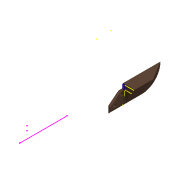
# Autodesk Inventor part: encoder guard mirror
Saved by Autodesk Inventor 2020 (Build 240168000, 168)
## iProperties
Created: 2020-01-15
Part Number: encoder guard mirror
Material: Bronze, Cast
Document SubType Name: Modeling
Designer: ball
Density: 8.87 g/cm^3
Appearance: Bronze - Satin
Mass: 40.1382 g
Surface Area: 24.9444 cm^2
Volume: 4.52517 cm^3
Author: ball
Autodesk Inventor part; units mm, degrees
ref_plane "YZ Plane" through (0, 0, 0) normal (1, 0, 0) x (0, 1, 0)
ref_plane "XZ Plane" through (0, 0, 0) normal (0, 1, 0) x (-1, 0, 0)
ref_plane "XY Plane" through (0, 0, 0) normal (0, 0, 1) x (1, 0, 0)
ref_plane "Work Plane6" through (0, 0, 0) normal (0, 0, 1) x (1, 0, 0)
sketch "Sketch1" plane through (0, 0, 0) normal (0, 0, 1) x (1, 0, 0)
  line L0 (25.4, -44.45) -> (0, -44.45) construction
  line L1 (25.4, -44.45) -> (12.7, -44.45)
  line L2 (12.7, -65.151) -> (25.4, -44.45)
  line L3 (12.7, -44.45) -> (12.7, -65.151)
  point P0 (0, 0)
  dimension "d0" = 20.701
  dimension "d1" = 12.7
  constraints: 6 end point, 1 midpoint, 1 perpendicular, 1 point on line
  measures "d0" distance from line of L0 L2.start
  measures "d1" distance from line of L1.start L3
revolve "Revolution1" add sketch "Sketch1" angle 180 mid plane about axis through (25.4, -44.45, 0) along (-1, 0, 0)
ref_plane "Work Plane10" through (12.7, -44.45, -31.115) normal (0, -1, 0) x (0, 0, -1)
sketch "Sketch2" plane through (12.7, -44.45, -31.115) normal (0, -1, 0) x (0, 0, -1)
  line L0 (0.635, -12.7) -> (0.635, 12.7) construction
  line L1 (9.525, 12.7) -> (-9.525, 12.7) construction
  line L2 (0.635, 0) -> (-31.115, 0)
  line L3 (-31.115, 0) -> (-31.115, 12.7)
  line L4 (-31.115, 12.7) -> (0.635, 12.7)
  line L5 (0.635, 12.7) -> (0.635, 0)
  point P0 (-31.115, -12.7)
  constraints: 8 end point, 2 parallel, 1 horizontal, 1 midpoint, 1 perpendicular
extrude "Extrusion1" add sketch "Sketch2" along normal blind 5.08
sketch "Sketch3" plane through (12.7, -49.53, -31.115) normal (0, -1, 0) x (1, 0, 0)
  point P0 (-12.7, 31.115)
ref_plane "Work Plane9" through (25.4, -44.45, -31.75) normal (0, 0, -1) x (-1, 0, 0)
sketch "Sketch4" plane through (25.4, -44.45, -31.75) normal (0, 0, -1) x (-1, 0, 0)
  line L0 (12.7, -5.08) -> (3.1166, -5.08)
  line L1 (0, 0) -> (12.7, -20.701) projected
  line L2 (12.7, -20.701) -> (12.7, 0) projected
  line L3 (12.7, -5.08) -> (12.7, -20.701)
  line L4 (12.7, -20.701) -> (3.1166, -5.08)
  point P0 (25.4, 44.45)
  constraints: 6 end point, 1 collinear, 1 horizontal, 1 point on line
extrude "Extrusion2" add sketch "Sketch4" against normal through all
ref_plane "Work Plane8" through (25.4, -47.625, 0) normal (0, 0, 1) x (1, 0, 0)
sketch "Sketch5" plane through (25.4, -47.625, 0) normal (0, 0, 1) x (1, 0, 0)
  line L0 (-12.7, 3.175) -> (0, 3.175) projected
  line L1 (-3.6741, -2.8138) -> (0, 3.175) projected
  line L2 (0, 3.175) -> (-3.6741, -2.8138)
  line L3 (-3.6741, -2.8138) -> (0, -4.7625)
  line L4 (0, -4.7625) -> (4.0347, 1.814)
  line L5 (4.0347, 1.814) -> (0, 3.175)
  point P0 (-25.4, 47.625)
  constraints: 8 end point, 1 collinear, 1 parallel
extrude "Extrusion3" cut sketch "Sketch5" against normal through all
sketch "Sketch6" plane through (12.7, -44.45, 20.701) normal (0, 1, 0) x (1, 0, 0)
  line L0 (0, 0) -> (0, 52.451) projected
  point P0 (-12.7, 20.701)
ref_plane "Work Plane3" through (25.4, -44.45, -57.15) normal (0, 0, -1) x (-1, 0, 0)
mirror "Mirror1" about plane through (25.4, -44.45, -57.15) normal (0, 0, -1) of "Revolution1", "Extrusion1", "Extrusion2", "Extrusion3"
sketch "Sketch7" plane through (12.7, -65.151, 0) normal (0.8523757, -0.5229299, 0) x (0, 0, -1)
  line L0 (-47.625, 53.975) -> (53.975, 44.45)
  line L1 (53.975, 44.45) -> (52.3875, 4.7625)
  line L2 (52.3875, 4.7625) -> (38.1, -4.7625)
  line L3 (38.1, -4.7625) -> (-33.3375, -3.175)
  line L4 (-33.3375, -3.175) -> (-47.625, 53.975)
  point P0 (0, 48.8919)
  constraints: 10 end point
extrude "Extrusion4" cut sketch "Sketch7" against normal blind 254
sketch "Sketch8" plane through (12.7, -65.151, -82.55) normal (-1, 0, 0) x (0, 0, 1)
  line L0 (0, 20.701) -> (-52.451, 20.701) projected
  line L1 (0, 20.701) -> (-8.89, 20.701)
  line L2 (0, 20.701) -> (0, 0) projected
  arc A0 (-8.89, 20.701) -> (0, 7.9375) centre (-2.2225, 15.8673) ccw
  line L3 (-8.89, 20.701) -> (1.5875, 28.575)
  line L4 (1.5875, 28.575) -> (11.1125, 12.7)
  line L5 (11.1125, 12.7) -> (0, 7.9375)
  point P0 (82.55, 65.151)
  dimension "d13" = 8.89
  constraints: 8 end point, 2 point on circle, 2 point on line, 1 centre point
  measures "d13" distance of L0.start L1.end
extrude "Extrusion5" cut sketch "Sketch8" against normal blind 254 contours L2 A0 L0
sketch "Sketch9" plane through (12.7, -65.151, -114.3) normal (-1, 0, 0) x (0, 0, 1)
  arc A0 (22.86, 20.701) -> (31.75, 7.9375) centre (29.5275, 15.8673) ccw projected
  line L0 (21.2988, 15.5377) -> (21.2988, 22.6528)
  line L1 (21.2988, 22.6528) -> (30.1625, 22.225)
  line L2 (30.1625, 22.225) -> (26.9875, 14.2875)
  line L3 (26.9875, 14.2875) -> (21.2988, 15.5377)
  point P0 (114.3, 65.151)
  constraints: 8 end point, 1 point on circle, 1 vertical
extrude "Extrusion6" cut sketch "Sketch9" against normal through all contours L0 L1 L2 L3
sketch "Sketch10" plane through (12.7, -65.151, -114.3) normal (-1, 0, 0) x (0, 0, 1)
  arc A0 (21.2988, 16.1968) -> (31.75, 7.9375) centre (29.5275, 15.8673) ccw projected
  line L0 (29.3335, 7.6342) -> (32.248, 7.6342)
  line L1 (32.248, 7.6342) -> (31.75, 7.9375)
  line L2 (31.75, 7.9375) -> (30.1625, 7.9375)
  line L3 (30.1625, 7.9375) -> (29.3335, 7.6342)
  point P0 (114.3, 65.151)
  constraints: 8 end point, 1 horizontal, 1 point on circle
extrude "Extrusion7" cut sketch "Sketch10" against normal blind 254
sketch "Sketch11" plane through (12.7, -57.5168, -82.55) normal (0, 0, 1) x (1, 0, 0)
  line L0 (0, -7.6342) -> (0, 13.0668) projected
  line L1 (9.9367, 8.5626) -> (4.6822, -0.0023) projected
  line L2 (0, -7.6342) -> (4.6822, -0.0023)
  line L3 (4.6836, 0) -> (0, 0) projected
  line L4 (4.6822, -0.0023) -> (0, 0)
  line L5 (0, 0) -> (0, -7.6342)
  point P0 (-12.7, 57.5168)
  constraints: 6 end point, 1 collinear
extrude "Extrusion8" add sketch "Sketch11" along normal blind 5.08 contours L0 L4 L2
sketch "Sketch12" plane through (12.7, -48.9542, -93.0012) normal (-1, 0, 0) x (0, 0, 1)
  circle A0 centre (10.756, -9.9738) radius 1.9304
  line L0 (15.5312, -8.5626) -> (15.5312, -16.1968) projected
  line L1 (-21.2988, -16.1968) -> (15.5312, -16.1968) projected
  point P0 (93.0012, 48.9542)
  dimension "d22" = 3.8608
  dimension "d23" = 4.7752
  dimension "d24" = 6.223
  constraints: 1 centre point
  measures "d22" diameter of A0
  measures "d23" distance from line of L0 A0.centre
  measures "d24" distance from line of L1 A0.centre
sketch "Sketch13" plane through (12.7, -48.9542, -93.0012) normal (-1, 0, 0) x (0, 0, 1)
  line L0 (10.4512, -8.5649) -> (15.5312, -8.5649) projected
  line L1 (15.5312, -8.5649) -> (15.5312, -6.1368)
  line L2 (15.5312, -6.1368) -> (-2.8039, -6.1368)
  line L3 (-2.8039, -6.1368) -> (-1.5875, -14.2875)
  line L4 (-1.5875, -14.2875) -> (15.5312, -14.2875)
  line L5 (15.5312, -8.5626) -> (15.5312, -16.1968) projected
  point P0 (93.0012, 48.9542)
  constraints: 8 end point, 1 horizontal, 1 perpendicular, 1 point on line, 1 vertical
extrude "Extrusion9" add sketch "Sketch13" against normal blind 12.7
sketch "Sketch14" plane through (12.7, -57.5168, -77.47) normal (0, 0, 1) x (1, 0, 0)
  line L0 (0, -7.6342) -> (0, 13.0668) projected
  line L1 (0, -7.6342) -> (7.3478, 4.3426)
  line L2 (9.9367, 8.5626) -> (6.1718, 2.4257) projected
  line L3 (17.4483, 5.0236) -> (19.05, -6.35)
  line L4 (19.05, -6.35) -> (0, -7.6342)
  line L5 (17.4483, 5.0236) -> (7.3478, 4.3426)
  point P0 (-12.7, 57.5168)
  constraints: 8 end point, 1 parallel, 1 point on line
extrude "Extrusion10" cut sketch "Sketch14" against normal through all
fillet "Fillet2" radius 3.175 1 edges at (15.7859, -55.091, -90.6117)
extrude "Extrusion11" cut sketch "Sketch12" against normal blind 12.7
sketch "Sketch15" plane through (12.7, -57.5168, -77.47) normal (0, 0, 1) x (1, 0, 0)
  point P0 (-12.7, 57.5168)
sketch "Sketch16" plane through (12.7, -57.5168, -77.47) normal (0, 0, 1) x (1, 0, 0)
  line L0 (0, 2.4257) -> (6.1718, 2.4257) projected
  line L1 (6.1718, 2.4257) -> (2.4532, 2.4257)
  line L2 (2.4532, 2.4257) -> (2.4532, -6.1097)
  line L3 (2.4532, -6.1097) -> (7.9375, -4.7625)
  line L4 (0, 2.4257) -> (6.1718, 2.4257) projected
  line L5 (7.9375, -4.7625) -> (6.1718, 2.4257)
  point P0 (-12.7, 57.5168)
  constraints: 8 end point, 2 perpendicular, 1 point on line
extrude "Extrusion12" cut sketch "Sketch16" against normal blind 8.89
sketch "Sketch17" plane through (12.7, -57.5168, -77.47) normal (0, 0, 1) x (1, 0, 0)
  line L0 (0, 2.4257) -> (6.1718, 2.4257) projected
  line L1 (0, 2.4257) -> (0, 8.53)
  line L2 (0, -7.6342) -> (0, 13.0668) projected
  line L3 (9.9367, 8.5626) -> (0, 8.5626) projected
  line L4 (9.9367, 8.5626) -> (6.1718, 2.4257)
  line L5 (9.9367, 8.5626) -> (7.1064, 3.9492) projected
  line L6 (6.1718, 2.4257) -> (9.9367, 8.5626)
  line L7 (0, -7.6342) -> (0, 2.4257) projected
  line L8 (0, 8.5626) -> (0, 2.4257)
  line L9 (0, 2.4257) -> (0, 8.5626)
  point P0 (-12.7, 57.5168)
  constraints: 10 end point, 4 collinear, 1 point on line
extrude "Extrusion13" add sketch "Sketch17" against normal through all
sketch "Sketch18" plane through (12.7, -57.5168, -77.47) normal (0, 0, 1) x (1, 0, 0)
  line L0 (2.4532, 2.4257) -> (6.1718, 2.4257) projected
  line L1 (2.4532, 2.4257) -> (2.4532, 8.5626)
  line L2 (9.9367, 8.5626) -> (0, 8.5626) projected
  line L3 (6.1718, 2.4257) -> (9.9367, 8.5626) projected
  line L4 (2.4532, 8.5626) -> (9.9367, 8.5626)
  line L5 (9.9367, 8.5626) -> (6.1718, 2.4257)
  line L6 (2.4532, -3.6355) -> (2.4532, 2.4257) projected
  line L7 (6.1718, 2.4257) -> (2.4532, 2.4257)
  point P0 (-12.7, 57.5168)
  constraints: 8 end point, 1 collinear, 1 horizontal, 1 parallel, 1 point on line, 1 vertical
extrude "Extrusion14" cut sketch "Sketch18" against normal blind 15.494
sketch "Sketch19" plane through (15.1532, -61.1523, -77.47) normal (1, 0, 0) x (0, 0, -1)
  circle A0 centre (12.7, 8.9553) radius 1.9304
  line L0 (36.83, -3.9987) -> (0, -3.9987) projected
  line L1 (0, 0) -> (0, 12.1981) projected
  point P0 (-77.47, 61.1523)
  dimension "d38" = 3.8608
  dimension "d39" = 12.954
  dimension "d40" = 12.7
  constraints: 1 centre point
  measures "d38" diameter of A0
  measures "d39" distance from line of L0 A0.centre
  measures "d40" distance from line of L1 A0.centre
extrude "Extrusion15" cut sketch "Sketch19" against normal blind 15.494
sketch "Sketch20" plane through (15.1532, -61.1523, -77.47) normal (1, 0, 0) x (0, 0, -1)
  line L0 (0, 12.1981) -> (15.5312, 12.1981) projected
  line L1 (11.363, 12.1981) -> (0, 3.175)
  line L2 (0, 3.175) -> (-1.5875, 9.525)
  line L3 (-1.5875, 9.525) -> (0, 16.13)
  line L4 (0, 16.13) -> (11.363, 12.1981)
  point P0 (-77.47, 61.1523)
  constraints: 8 end point, 1 point on line
extrude "Extrusion16" cut sketch "Sketch20" against normal blind 15.494
sketch "Sketch21" plane through (15.1532, -61.1523, -77.47) normal (1, 0, 0) x (0, 0, -1)
  line L0 (11.363, 12.1981) -> (15.494, 12.1981) projected
  line L1 (13.9508, 12.1981) -> (10.6034, 11.5949)
  line L2 (11.363, 12.1981) -> (0, 3.175) projected
  line L3 (10.6034, 11.5949) -> (9.2319, 13.3221)
  line L4 (9.2319, 13.3221) -> (12.7, 14.2875)
  line L5 (12.7, 14.2875) -> (13.9508, 12.1981)
  point P0 (-77.47, 61.1523)
  constraints: 8 end point, 2 point on line, 1 perpendicular
extrude "Extrusion17" cut sketch "Sketch21" against normal blind 15.494
sketch "Sketch22" plane through (12.7, -44.45, -93.0012) normal (0, 0, 1) x (1, 0, 0)
  line L0 (0, -4.5042) -> (2.4532, -4.5042) projected
  line L1 (0, -4.5042) -> (2.4532, -4.5042)
  line L2 (2.4532, -4.5042) -> (2.4532, 0)
  line L3 (0, 0) -> (12.7, 0) projected
  line L4 (2.4532, 0) -> (0, 0)
  line L5 (0, -20.701) -> (0, 0) projected
  line L6 (0, 0) -> (0, -4.5042)
  line L7 (2.4532, -4.5042) -> (9.9367, -4.5042) projected
  line L8 (0, -4.5042) -> (2.4532, -4.5042)
  line L9 (2.4532, -4.5042) -> (0, -4.5042)
  line L10 (0, -5.1073) -> (0, -4.5042) projected
  line L11 (0, -4.5042) -> (2.4532, -4.5042)
  point P0 (-12.7, 44.45)
  constraints: 14 end point, 3 collinear, 2 horizontal, 2 perpendicular, 1 point on line
sketch "Sketch23" plane through (12.7, -44.45, -93.0012) normal (0, 0, 1) x (1, 0, 0)
  line L0 (2.4532, -5.1073) -> (0, -5.1073) projected
  line L1 (0, -20.701) -> (0, 0) projected
  line L2 (0, -5.1073) -> (0, 0)
  line L3 (0, 0) -> (2.4532, 0)
  line L4 (2.4532, -10.641) -> (2.4532, -4.5042) projected
  line L5 (2.4532, 0) -> (2.4532, -5.1073)
  line L6 (2.4532, -4.5042) -> (9.9367, -4.5042) projected
  line L7 (2.4532, -5.1073) -> (0, -5.1073)
  point P0 (-12.7, 44.45)
  constraints: 8 end point, 3 perpendicular, 1 vertical
sketch "Sketch24" plane through (15.1532, -61.1523, -77.47) normal (1, 0, 0) x (0, 0, -1)
  line L0 (13.9508, 12.1981) -> (10.6034, 11.5949) projected
  line L1 (10.6034, 11.5949) -> (11.7393, 12.1981)
  line L2 (11.7393, 12.1981) -> (13.9508, 12.1981)
  line L3 (13.9508, 12.1981) -> (10.6034, 11.5949)
  point P0 (-77.47, 61.1523)
  constraints: 6 end point, 1 horizontal
extrude "Extrusion18" add sketch "Sketch24" against normal up to surface (2.4532 mm away)
sketch "Sketch25" plane through (12.7, -57.5168, -86.36) normal (0, 0, 1) x (1, 0, 0)
  line L0 (9.9367, 8.5626) -> (6.1718, 2.4257) projected
  line L1 (6.1718, 2.4257) -> (2.4532, 2.4257) projected
  line L2 (6.1718, 2.4257) -> (2.4532, 2.4257)
  line L3 (6.1718, 2.4257) -> (2.4532, -3.6355) projected
  line L4 (2.4532, 2.4257) -> (2.4532, -3.6355)
  line L5 (2.4532, -3.6355) -> (6.1718, 2.4257)
  point P0 (-12.7, 57.5168)
  constraints: 6 end point, 2 collinear, 1 perpendicular
extrude "Extrusion19" cut sketch "Sketch25" against normal blind 6.604
sketch "Sketch26" plane through (12.7, -57.5168, -77.47) normal (0, 0, 1) x (1, 0, 0)
  line L0 (0, 8.5626) -> (0, 13.0668) projected
  line L1 (0, 8.5626) -> (0, 13.0668)
  line L2 (0, 13.0668) -> (12.7, 13.0668) projected
  line L3 (0, 13.0668) -> (12.7, 13.0668)
  line L4 (12.7, 13.0668) -> (2.4532, -3.6355)
  line L5 (0, -7.6342) -> (12.7, 13.0668) projected
  line L6 (2.4532, 8.5626) -> (2.4532, 7.9594) projected
  line L7 (2.4532, 8.5626) -> (0, 8.5626)
  line L8 (2.4532, 8.5626) -> (2.4532, -3.6355)
  point P0 (-12.7, 57.5168)
  constraints: 10 end point, 2 vertical, 1 collinear, 1 perpendicular, 1 point on line
extrude "Extrusion20" cut sketch "Sketch26" against normal blind 16.51
ref_plane "Work Plane4" through (0, 0, -114.3) normal (0, 0, 1) x (1, 0, 0)
ref_plane "Work Plane5" through (12.7, -44.45, -83.185) normal (0, 1, 0) x (0, 0, 1)
body "Solid1"
